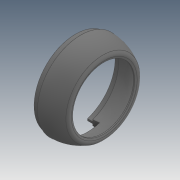
# Autodesk Inventor part: cover2
Saved by Autodesk Inventor 2020.3 (Build 243373000, 373)
## iProperties
Created: 2021-01-25
Part Number: cover2
Material: Generic
Document SubType Name: Modeling
Designer: serge
Density: 1 g/cm^3
Appearance: Gray
Sheet Metal Rule: Default
Author: serge
Autodesk Inventor part; units mm, degrees
ref_plane "YZ Plane" through (0, 0, 0) normal (1, 0, 0) x (0, 1, 0)
ref_plane "XZ Plane" through (0, 0, 0) normal (0, 1, 0) x (-1, 0, 0)
ref_plane "XY Plane" through (0, 0, 0) normal (0, 0, 1) x (1, 0, 0)
sketch "Sketch1" plane through (0, 0, 0) normal (1, 0, 0) x (0, 1, 0)
  circle A0 centre (0, 0) radius 25
  circle A1 centre (0, 0) radius 22
  line L0 (25, 0) -> (-25, 0)
  point P0 (-22, 0)
  point P1 (22, 0)
  dimension "d0" = 50
  dimension "d1" = 3
  constraints: 2 centre point, 2 coincident, 2 end point, 2 point on circle, 1 horizontal
  measures "d0" diameter of A0
  measures "d1" radial gap between concentric circles of A0 A1
revolve "Revolution1" add sketch "Sketch1" angle 360 about axis through (0, 25, 0) along (0, -1, 0) picked at (23.7578, -1.9943) contours A0 L0 A1
split "Split1" plane through (0, 0, 0) removes the side toward (-1, 0, 0)
sketch "Sketch8" plane through (0, 0, 0) normal (-1, 0, 0) x (0, 0, 1)
  circle A0 centre (0, 0) radius 18
  dimension "d40" = 36
  constraints: 1 centre point, 1 coincident
  measures "d40" diameter of A0
extrude "Extrusion7" cut sketch "Sketch8" against normal blind 39
chamfer "Chamfer1" distance 4 angle 45 1 edges at (17.3494, -0.0007, -18)
sketch "Sketch9" plane through (0, 0, 0) normal (-1, 0, 0) x (0, 0, 1)
  circle A0 centre (0, 0) radius 24
  circle A1 centre (0, 0) radius 23
  dimension "d46" = 48
  dimension "d47" = 1
  constraints: 2 centre point, 2 coincident
  measures "d46" diameter of A0
  measures "d47" radial gap between concentric circles of A0 A1
extrude "Extrusion8" add sketch "Sketch9" along normal blind 3
sketch "Sketch10" plane through (0, 0, 0) normal (-1, 0, 0) x (0, 0, 1)
  line L0 (0, 0) -> (0, -25)
  circle A0 centre (0, 0) radius 25
  line L1 (7, -17.5) -> (-7, -17.5)
  line L2 (-7, -17.5) -> (-7, -32.5)
  line L3 (-7, -32.5) -> (7, -32.5)
  line L4 (7, -32.5) -> (7, -17.5)
  line L5 (7, -17.5) -> (-7, -32.5) construction
  line L6 (-7, -17.5) -> (7, -32.5) construction
  dimension "d50" = 14
  dimension "d51" = 15
  constraints: 14 end point, 2 midpoint, 2 parallel, 1 horizontal, 1 perpendicular, 1 vertical, 1 vertical alignment, 2 other
  measures "d50" distance of L2.end L3.end
  measures "d51" distance of L3.end L1.start
extrude "Extrusion9" cut sketch "Sketch10" along normal mid plane 8 contours L1 L4 A0 L0 | L0 A0 L2 L1 | A0 L4 L3 L2
fillet "Fillet1" radius 2 1 edges at (14.2565, -0.0008, -20.5366)
body "Solid1"
